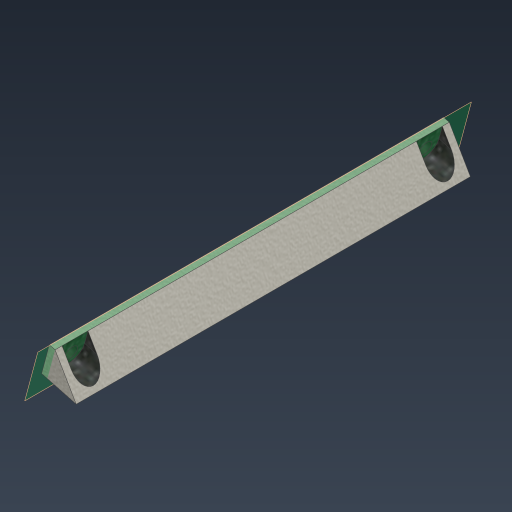
# Autodesk Inventor part: plog
Saved by Autodesk Inventor 2023 (Build 270158000, 158)
## iProperties
Created: 2025-03-31
Part Number: plog
Material: Steel
Document SubType Name: Modeling
Designer: szymo
Density: 7.85 g/cm^3
Appearance: Plate
Mass: 30.6003 g
Surface Area: 29.108 cm^2
Volume: 3.89813 cm^3
Author: szymo
Autodesk Inventor part; units mm, degrees
ref_plane "YZ Plane" through (0, 0, 0) normal (1, 0, 0) x (0, 1, 0)
ref_plane "XZ Plane" through (0, 0, 0) normal (0, 1, 0) x (-1, 0, 0)
ref_plane "XY Plane" through (0, 0, 0) normal (0, 0, 1) x (1, 0, 0)
sketch "Sketch1" plane through (0, 0, 0) normal (0, 0, 1) x (1, 0, 0)
  line L0 (-88.5894, 124.481) -> (10.4106, 124.481) construction
  line L1 (10.4106, -13.8838) -> (3.1661, -11.9426)
  line L2 (3.1661, -11.9426) -> (5.1073, -4.6982)
  line L3 (5.1073, -4.6982) -> (10.4106, -13.8838)
  line L4 (6.0732, -4.957) -> (5.1073, -4.6982)
  line L5 (5.1073, -4.6982) -> (3.5544, -10.4937)
  line L6 (3.5544, -10.4937) -> (4.5203, -10.7526)
  line L7 (4.5203, -10.7526) -> (6.0732, -4.957)
  line L8 (5.1073, -4.6982) -> (3.6584, -4.31)
  line L9 (3.6584, -4.31) -> (1.7173, -11.5544)
  line L10 (1.7173, -11.5544) -> (3.1661, -11.9426)
  line L11 (1.3286, 24.5015) -> (4.9073, -4.6446)
  line L12 (4.9073, -4.6446) -> (2.801, -3.9014)
  line L13 (2.801, -3.9014) -> (-0.6853, 24.4925)
  line L14 (-0.6853, 24.4925) -> (1.3286, 24.5015)
  line L15 (-65.1645, -13.8838) -> (10.4106, -13.8838) construction
  line L16 (10.4106, -13.8838) -> (10.4106, 124.481) construction
  circle A0 centre (-70.7481, 2.6162) radius 12.5
  circle A1 centre (-45.2483, 2.7295) radius 12.5
  line L17 (-70.7481, -9.8838) -> (-41.2673, -9.8838) construction
  line L18 (0.8562, 1.8179) -> (0.8095, 12.3178)
  line L19 (5.1073, -4.6982) -> (4.9073, -4.6446) construction
  line L20 (-88.0263, -2.3268) -> (-88.1614, 28.1041)
  line L21 (-86.1615, 28.113) -> (-88.1614, 28.1041)
  point P0 (0.8318, 7.2969)
  point P1 (0.8339, 6.8388)
  dimension "d0" = 99
  dimension "d4" = 90
  dimension "d5" = 45
  dimension "d6" = 7.5
  dimension "d8" = 1
  dimension "d10" = 0
  dimension "d11" = 1.5
  dimension "d13" = 75
  dimension "d15" = 2
  dimension "d17" = 6
  dimension "d18" = 83
  dimension "d19" = 15
  dimension "d22" = 4
  dimension "d27" = 0.1
  dimension "d28" = 0.2
  dimension "d29" = 4
  constraints: 42 end point, 5 point on line, 4 horizontal, 3 parallel, 3 perpendicular, 1 centre point, 1 coincident, 1 vertical, 1 vertical alignment, 20 other
  measures "d0" distance of L0.start L0.end
  measures "d4" angle of L1 L2
  measures "d5" angle of L1 L3
  measures "d6" distance of L1.end L2.end
  measures "d8" distance of L6.end L6.start
  measures "d10" distance from line of L2 L4.end
  measures "d11" distance of L2.end L8.end
  measures "d13" angle of L0 L9
  measures "d15" distance between parallel lines of L11 L13
  measures "d17" distance of L6.end L4.start
  measures "d18" angle of L0 L13
  measures "d19" angle of L15 L1
  measures "d22" distance between parallel lines of L17 L15
  measures "d27" distance from line of L12 L8.end
  measures "d28" horizontal distance of L4.end L11.end
  measures "d29" distance between parallel lines of L21 L14
ref_plane "Work Plane1" through (-31.6, -3, -99) normal (0, 0, -1) x (0, 1, 0)
extrude "Extrusion1" add sketch "Sketch1" against normal up to surface (99 mm away) contours L1 L2 L6 L7 L3 | L10 L9 L8 L2 | L7 L6 L2 L3
ref_plane "Work Plane2" through (5.1073, -4.6982, 0) normal (-0.9659258, 0.258819, 0) x (0, 0, 1)
sketch "Sketch2" plane through (5.1073, -4.6982, 0) normal (-0.9659258, 0.258819, 0) x (0, 0, 1)
  line L0 (0, -7.5) -> (-10, -7.5)
  line L1 (0, -7.5) -> (0, 0)
  line L2 (-10, 0) -> (-10, -7.5)
  line L3 (0, 0) -> (-10, 0)
  circle A0 centre (-5, -3.25) radius 3.25
  line L4 (0, 0) -> (0, -7.5) projected
  line L5 (0, 0) -> (-10, -7.5) construction
  line L6 (-10, 0) -> (0, -7.5) construction
  line L7 (-5, -3.75) -> (-5, -3.25) construction
  line L8 (-1.75, -3.25) -> (-1.75, 0)
  line L9 (-8.25, -3.25) -> (-8.25, 0)
  line L10 (-99, -7.5) -> (-89, -7.5)
  line L11 (-89, 0) -> (-89, -7.5)
  line L12 (-99, -7.5) -> (-99, 0)
  line L13 (-99, 0) -> (-89, 0)
  line L14 (0, -7.5) -> (-99, -7.5) projected
  line L15 (-89, 0) -> (-99, -7.5) construction
  line L16 (-99, 0) -> (-99, -7.5) projected
  line L17 (-89, -7.5) -> (-99, 0) construction
  circle A1 centre (-94, -3.25) radius 3.25
  line L18 (-94, -3.75) -> (-94, -3.25) construction
  line L19 (-90.75, -3.25) -> (-90.75, 0)
  line L20 (-97.25, -3.25) -> (-97.25, 0)
  line L21 (0, 0) -> (-99, 0) projected
  point P0 (0, 3.2162)
  dimension "d30" = 6.5
  dimension "d41" = 6.5
  constraints: 36 end point, 6 tangent, 6 vertical, 4 horizontal, 4 perpendicular, 4 point on circle, 4 point on line, 2 centre point, 2 midpoint, 1 coincident, 8 other
  measures "d30" diameter of A0
  measures "d41" diameter of A1
extrude "Extrusion2" cut sketch "Sketch2" against normal through all contours L8 A0 L3 | L3 A0 L9 | A0 | L19 A1 L13 | A1 L20 L13 | A1
hole "Hole1" at (4.1367, -8.3204, -5) at (4.1367, -8.3204, -94) direction (-0.9659258, 0.258819, 0) diameter 3.2 end through all clearance for "Countersunk Flat Head Screw ISO 2009/7046" size "M3" standard "ISO"
body "Solid1"
